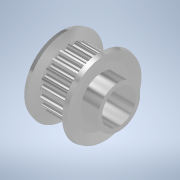
# Autodesk Inventor part: pulley
Saved by Autodesk Inventor 2020 (Build 240168000, 168)
## iProperties
Part Number: pulley
Material: Aluminum 6061
Catalog Web Link: www.cadenas.de
Description: GPA__GT2040, GPA__GT2060, GPA__GT2090_body-High Torque Timing Pulleys 2GT Type
Vendor: MISUMI
Document SubType Name: Modeling
Designer: partserver
Manufacturer: MISUMI
Mass: 2.85895 g
Surface Area: 16.6375 cm^2
Volume: 1.05887 cm^3
Density: 2.7 g/cm^3
Appearance: Aluminum - Flat
Category: PARTsolutions
Company: MISUMI
PSOL_IDENT_0: {$CADENAS_DATA\23d-libs\misumi\metric\51_timing_pulleys\gpa__gt2\gpa_gt2.prj},382 {VTYP=3D},{NB=GPA2
PSOL_IDENT_1: 2GT2060-A-H6_b},{LINA=GPA22GT2060-A-H6},{NN=GPA__GT2040, GPA__GT2060, GPA__GT2090_body},{DATE=17.01.
PSOL_IDENT_2: 2019 09:47:54},{GEOMDATE=17.12.2018 08:21:00},{VERSION=},{LINEID=60},{WBVAR=TNW,PS,SBS,DD,Z,J,Q,R,S,
PSOL_IDENT_3: T,ALT1,ALT2,M,QSC,QFC,QTC,ALT3,K,KSC,KFC,KTC,ALT4,ZM,ZSC,ZFC,ZTC,ALT5,BC,ALT6,ALT7,ALT8,FC},{WBNUMER
PSOL_IDENT_4: IC=DD,Z,J,Q,R,S,T,QSC,QFC,QTC,K,KSC,KFC,KTC,ZSC,ZFC,ZTC,BC,FC}  {NB=GPA22GT2060-A-H6_b},{LINA=GPA22G
PSOL_IDENT_5: T2060-A-H6},{KT=DUMMY},{PN=GPA22GT2060-A-H6},{TYPE=GPA},{NT=22},{TNW=GT2060},{BW=6},{A=7.0},{W=10.3}
PSOL_IDENT_6: ,{L=18.0},{PS=A},{PSA= 'A','B' },{SBS=H},{SBSALG= 'H','Round Hole','V','Stepped Hole','Y','Both Ends
PSOL_IDENT_7: Stepped Hole' },{DD=6.00},{DDALG=[4:4/1],[4.5],[5:6/1]},{DDHA=[4:4/1],[4.5],[5:6/1]},{DDHB=[4:4/1]}
PSOL_IDENT_8: ,{DDPA=},{DDPB=},{DDNA=},{DDNB=},{DDNKA=0},{DDNKB=0},{DDVA=[4:4/1]},{DDVFB=},{DDYA=[4:4/1]},{Z=0},{Z
PSOL_IDENT_9: ALG=0},{ZMIN=8},{ZAMAX=6},{ZBMAX=0},{J=0.0},{JALG=0},{JMAX=8.3},{Q=0},{R=0},{QRALG=0},{QRMIN=8},{QRM
PSOL_IDENT_10: AX=6},{S=0.0},{SALG=0},{SMAX=4.300},{T=0.0},{TALG=0},{TMAX=5.000},{PD=14.01},{OD=13.50},{D=8},{DE=10
PSOL_IDENT_11: },{DDZ=6},{F=18},{E=10},{BB=0},{TT=0},{M1=4},{AC=-},{ALT1=},{ALT1A= '','Not applicable' },{ANG=114.5
PSOL_IDENT_12: 45455},{ALT2=},{ALT2A= '','Not applicable' },{M=N/A},{MALG= 'N/A' },{MM=0.000},{MPHD=0.000},{MA= 'N/
PSOL_IDENT_13: A' },{MSA= 'N/A' },{QSC=0.0},{QSCA=0},{QFC=0.0},{QFCA=0},{QTC=0.0},{QTCA=0},{QPCDMIN=10},{QPCDMINALG=
PSOL_IDENT_14: 10},{QPCDMAX=6},{ALT2PN=},{ALT3=},{ALT3A= '','Not applicable' },{K=0.0},{KA=0},{KAMIN=4},{KAMAX=0},{
PSOL_IDENT_15: KSMAX=0},{KSC=0.0},{KSCA=0},{KFC=0.0},{KFCA=0},{KTC=0.0},{KTCA=0},{KSCMIN=10.000},{KPCDMIN=10.000},{
PSOL_IDENT_16: KPCDMINALG=14.000},{KPCDMAX=6.000},{ALT3PN=},{ALT4=},{ALT4ALG= '','Not applicable' },{ALT4MIN=16.500
PSOL_IDENT_17: },{ALT4MAX=-0.500},{ZM=N/A},{ZMALG= 'N/A' },{ZMFTALG= 'N/A' },{ZMSALG= 'N/A' },{ZMDD1=0.0},{ZMDD2=0.
PSOL_IDENT_18: 0},{ZMHH=0.0},{ZSC=0.0},{ZSCALG=[0]},{ZFC=0.0},{ZFCALG=[0]},{ZTC=0.0},{ZTCALG=[0]},{ZPCDMIN=0.000},{
PSOL_IDENT_19: ZPCDMINALG=0.000},{ZPCDMAX=6.000},{ALT4PN=},{ALT5=},{ALT5ALG= '','Not applicable' },{ALT5PN=},{BC=0.
PSOL_IDENT_20: 0},{BCALG=0},{BCMIN=3.000},{BCMAX=7.700},{ALT6=},{ALT7=},{ALT7ALG= '','w/o Flange Attached on One Si
PSOL_IDENT_21: de Only','-RFC','with RFC (Flange Attached on The Boss Side Only)','-LFC','with LFC (Flange Attached
PSOL_IDENT_22: on The Opposite Side Only)' },{ALT8=},{ALT8ALG='','w/o FC (Flange Cut)','-FC','with FC (Flange Cut)'
PSOL_IDENT_23: },{ALT8PN=},{FC=0.0},{FCA=0},{ODAINT=16.500},{FCMIN=14.5},{FCMAX=16},{WLBC=10.3},{SL=3},{SL2=3},{KTT=
PSOL_IDENT_24: 3},{KYY=3.75},{TAP=0}
NB: GPA22GT2060-A-H6_b
NN: GPA__GT2040, GPA__GT2060, GPA__GT2090_body
NT: 22
NBSYN: $PN._b
LINA: GPA22GT2060-A-H6
CATALOG: Misumi
PN: GPA22GT2060-A-H6
TNW: GT2060
A: 7
W: 10.3
L: 18
PS: A
SBS: Round Hole
DD: 6
Z: 0
J: 0
Q: 0
R: 0
S: 0
T: 0
PD: 14.01
OD: 13.5
D: 8
F: 18
E: 10
AC: -
ALT1: Not applicable
ALT2: Not applicable
M: N/A
QSC: 0
QFC: 0
QTC: 0
ALT3: Not applicable
K: 0
KSC: 0
KFC: 0
KTC: 0
ALT4: Not applicable
ZM: N/A
ZMDD1: 0
ZMDD2: 0
ZMHH: 0
ZSC: 0
ZFC: 0
ZTC: 0
ALT5: Not applicable
BC: 0
ALT6: w/o Flange not Attached
ALT7: w/o Flange Attached on One Side Only
ALT8: w/o FC (Flange Cut)
FC: 0
SUPPLIER: MISUMI
ARTICLENO: GPA22GT2060-A-H6_b
BOMINFO: GPA22GT2060-A-H6
CREATOR: CADENAS GmbH
Title: GPA22GT2060-A-H6
Author: Cadenas PARTsolutions
Comments: High Torque Timing Pulleys 2GT Type
Autodesk Inventor part; units mm, degrees
ref_plane "YZ Plane" through (0, 0, 0) normal (1, 0, 0) x (0, 1, 0)
ref_plane "XZ Plane" through (0, 0, 0) normal (0, 1, 0) x (-1, 0, 0)
ref_plane "XY Plane" through (0, 0, 0) normal (0, 0, 1) x (1, 0, 0)
sketch "Sketch_16" plane through (0, 0, 0) normal (0, 0, 1) x (1, 0, 0)
  line L0 (5.15, 0) -> (-5.15, 0)
  line L1 (-5.15, 0) -> (-5.15, 5)
  line L2 (-5.15, 5) -> (-3.5, 5)
  line L3 (-3.5, 5) -> (-3.5, 6.75)
  line L4 (-3.5, 6.75) -> (3.5, 6.75)
  line L5 (3.5, 6.75) -> (3.5, 5)
  line L6 (3.5, 5) -> (5.15, 5)
  line L7 (5.15, 5) -> (5.15, 0)
  line L8 (5.15, 0) -> (-5.15, 0)
  constraints: 18 end point
revolve "Revolution1" add sketch "Sketch_16" angle 360 about axis through (5.15, 0, 0) along (1, 0, 0)
sketch "Sketch_18" plane through (0, 0, 0) normal (1, 0, 0) x (0, 1, 0)
  line L0 (6.9403, 0.9497) -> (6.6897, 0.9155)
  line L1 (6.6897, 0.9155) -> (6.7039, 0.7958)
  arc A0 (6.6046, 0.6712) -> (6.7039, 0.7958) centre (6.5927, 0.7826) ccw
  arc A1 (6.6046, 0.6712) -> (6.6046, -0.6712) centre (6.676, 0) ccw
  arc A2 (6.7039, -0.7958) -> (6.6046, -0.6712) centre (6.5927, -0.7826) ccw
  line L2 (6.7039, -0.7958) -> (6.6897, -0.9155)
  line L3 (6.6897, -0.9155) -> (6.9403, -0.9497)
  arc A3 (6.9403, -0.9497) -> (6.9403, 0.9497) centre (0, 0) ccw
  constraints: 8 end point, 8 point on circle, 4 centre point
extrude "Extrusion1" cut sketch "Sketch_18" along normal mid plane 7
pattern_circular "Circular Pattern1" count 22 over 360 about axis through (0, 0, 0) along (1, 0, 0) of "Extrusion1"
sketch "Sketch_20" plane through (0, 0, 0) normal (0, 0, 1) x (1, 0, 0)
  line L0 (50, 0) -> (-50, 0)
  line L1 (3.5, 6.75) -> (3.5, 5)
  line L2 (3.5, 5) -> (4.5, 5)
  line L3 (4.5, 5) -> (4.5, 6.6183)
  line L4 (4.5, 6.6183) -> (5.0688, 8.7412)
  line L5 (5.0688, 8.7412) -> (4.1029, 9)
  line L6 (4.1029, 9) -> (3.5, 6.75)
  constraints: 14 end point
revolve "Revolution2" add sketch "Sketch_20" angle 360 about axis through (50, 0, 0) along (1, 0, 0)
sketch "Sketch_21" plane through (0, 0, 0) normal (0, 0, 1) x (1, 0, 0)
  line L0 (50, 0) -> (-50, 0)
  line L1 (-5.0688, 8.7412) -> (-4.5, 6.6183)
  line L2 (-4.5, 6.6183) -> (-4.5, 5)
  line L3 (-4.5, 5) -> (-3.5, 5)
  line L4 (-3.5, 5) -> (-3.5, 6.75)
  line L5 (-3.5, 6.75) -> (-4.1029, 9)
  line L6 (-4.1029, 9) -> (-5.0688, 8.7412)
  constraints: 14 end point
revolve "Revolution3" add sketch "Sketch_21" angle 360 about axis through (50, 0, 0) along (1, 0, 0)
sketch "Sketch6" plane through (-5.15, 0, 0) normal (-1, 0, 0) x (0, 0, 1)
  circle A0 centre (0, 0) radius 4
  circle A1 centre (0, 0) radius 5
  dimension "d15" = 8
  constraints: 2 centre point, 2 coincident
  measures "d15" diameter of A0
extrude "Extrusion2" cut sketch "Sketch6" against normal blind 10.3 contours A0
extrude "Extrusion3" add sketch "Sketch6" along normal blind 3.35
body "Solid1"
